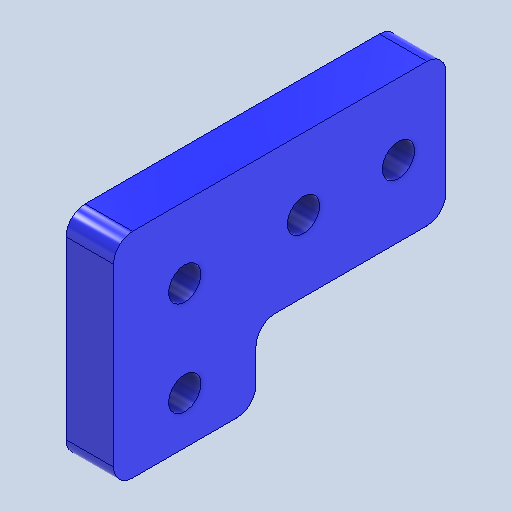
# Autodesk Inventor part: ball_loading_v1_Plate_ASP_F_2
Saved by Autodesk Inventor 2025.1 (Build 291241000, 241)
## iProperties
Created: 2024-11-12
Part Number: ball_loading_v1_Plate_ASP_F_2
Material: ABS プラスチック
Document SubType Name: Modeling
Designer: haruy
Density: 1.06 g/cm^3
Appearance: 青 - 壁塗料 - 光沢
Author: haruy
Autodesk Inventor part; units mm, degrees
ref_plane "YZ Plane" through (0, 0, 0) normal (1, 0, 0) x (0, 1, 0)
ref_plane "XZ Plane" through (0, 0, 0) normal (0, 1, 0) x (-1, 0, 0)
ref_plane "XY Plane" through (0, 0, 0) normal (0, 0, 1) x (1, 0, 0)
sketch "スケッチ1" plane through (0, 0, 0) normal (1, 0, 0) x (0, 1, 0)
  line L0 (-166.8338, 198.3583) -> (193.1662, 198.3583)
  line L1 (193.1662, 198.3583) -> (193.1662, 183.3583)
  line L2 (193.1662, 183.3583) -> (-166.8338, 183.3583)
  line L3 (-166.8338, 183.3583) -> (-166.8338, 198.3583)
  line L4 (-166.8338, 233.3583) -> (-181.8338, 233.3583)
  line L5 (-181.8338, 233.3583) -> (-181.8338, 5.8583)
  line L6 (-181.8338, 5.8583) -> (-166.8338, 5.8583)
  line L7 (-166.8338, 5.8583) -> (-166.8338, 233.3583)
  line L8 (-166.8338, 233.3583) -> (-181.8338, 233.3583)
  line L9 (-181.8338, 233.3583) -> (-181.8338, 218.3583)
  line L10 (-181.8338, 218.3583) -> (-166.8338, 218.3583)
  line L11 (-166.8338, 218.3583) -> (-166.8338, 233.3583)
  line L12 (-116.8338, 183.3583) -> (-101.8338, 183.3583)
  line L13 (-101.8338, 183.3583) -> (-101.8338, 5.8583)
  line L14 (-101.8338, 5.8583) -> (-116.8338, 5.8583)
  line L15 (-116.8338, 5.8583) -> (-116.8338, 183.3583)
  line L16 (193.1662, 183.3583) -> (178.1662, 183.3583)
  line L17 (178.1662, 183.3583) -> (178.1662, 5.8583)
  line L18 (178.1662, 5.8583) -> (193.1662, 5.8583)
  line L19 (193.1662, 5.8583) -> (193.1662, 183.3583)
  circle A0 centre (-141.8338, 138.3583) radius 12.5
  circle A1 centre (-141.8338, 98.3583) radius 18.75
  line L20 (193.1662, 5.8583) -> (-166.8338, 5.8583)
  line L21 (-181.8338, 158.3583) -> (-101.8338, 158.3583)
  line L22 (-101.8338, 78.3583) -> (-181.8338, 78.3583)
  circle A2 centre (-141.8338, 98.3583) radius 20
  line L23 (-124.3338, 198.3583) -> (-124.3338, 183.3583)
  line L24 (-101.8338, 183.3583) -> (-101.8338, 198.3583)
  line L25 (-146.8338, 198.3583) -> (-146.8338, 183.3583)
  line L26 (-166.8338, 205.8583) -> (-181.8338, 205.8583)
  line L27 (-166.8338, 175.8583) -> (-181.8338, 175.8583)
  circle A3 centre (158.1662, 138.3583) radius 12.5
  line L28 (193.1662, 163.3583) -> (178.1662, 163.3583)
  line L29 (170.6662, 198.3583) -> (170.6662, 183.3583)
  line L30 (-166.8338, -186.6417) -> (193.1662, -186.6417)
  line L31 (193.1662, -186.6417) -> (193.1662, -171.6417)
  line L32 (193.1662, -171.6417) -> (-166.8338, -171.6417)
  line L33 (-166.8338, -171.6417) -> (-166.8338, -186.6417)
  line L34 (-166.8338, -221.6417) -> (-181.8338, -221.6417)
  line L35 (-181.8338, -221.6417) -> (-181.8338, 5.8583)
  line L36 (-166.8338, 5.8583) -> (-166.8338, -221.6417)
  line L37 (-166.8338, -221.6417) -> (-181.8338, -221.6417)
  line L38 (-181.8338, -221.6417) -> (-181.8338, -206.6417)
  line L39 (-181.8338, -206.6417) -> (-166.8338, -206.6417)
  line L40 (-166.8338, -206.6417) -> (-166.8338, -221.6417)
  line L41 (-116.8338, -171.6417) -> (-101.8338, -171.6417)
  line L42 (-101.8338, -171.6417) -> (-101.8338, 5.8583)
  line L43 (-116.8338, 5.8583) -> (-116.8338, -171.6417)
  line L44 (193.1662, -171.6417) -> (178.1662, -171.6417)
  line L45 (178.1662, -171.6417) -> (178.1662, 5.8583)
  line L46 (193.1662, 5.8583) -> (193.1662, -171.6417)
  circle A4 centre (-141.8338, -126.6417) radius 12.5
  circle A5 centre (-141.8338, -86.6417) radius 18.75
  line L47 (-181.8338, -146.6417) -> (-101.8338, -146.6417)
  line L48 (-101.8338, -66.6417) -> (-181.8338, -66.6417)
  circle A6 centre (-141.8338, -86.6417) radius 20
  line L49 (-124.3338, -186.6417) -> (-124.3338, -171.6417)
  line L50 (-101.8338, -171.6417) -> (-101.8338, -186.6417)
  line L51 (-146.8338, -186.6417) -> (-146.8338, -171.6417)
  line L52 (-166.8338, -194.1417) -> (-181.8338, -194.1417)
  line L53 (-166.8338, -164.1417) -> (-181.8338, -164.1417)
  circle A7 centre (158.1662, -126.6417) radius 12.5
  line L54 (193.1662, -151.6417) -> (178.1662, -151.6417)
  line L55 (170.6662, -186.6417) -> (170.6662, -171.6417)
  line L56 (193.1662, 158.3583) -> (145.6662, 158.3583)
  line L57 (145.6662, 158.3583) -> (145.6662, 78.3583)
  line L58 (145.6662, 78.3583) -> (193.1662, 78.3583)
  line L59 (193.1662, 78.3583) -> (193.1662, 158.3583)
  line L60 (178.1662, 158.3583) -> (154.1437, 150.1934)
  line L61 (147.3229, 132.1397) -> (178.1662, 78.3583)
  circle A8 centre (-119.3338, 190.8583) radius 1.7
  circle A9 centre (-109.3338, 190.8583) radius 1.7
  circle A10 centre (-109.3338, 178.3583) radius 1.7
  circle A11 centre (-109.3338, 168.3583) radius 1.7
  line L62 (-101.8338, 163.3583) -> (-116.8338, 163.3583)
  point P0 (0, 0)
  point P1 (-174.3338, 200.8583)
  point P2 (-174.3338, 190.8583)
  point P3 (-174.3338, 180.8583)
  point P4 (-161.8338, 190.8583)
  point P5 (-151.8338, 190.8583)
  point P6 (185.6662, 178.3583)
  point P7 (185.6662, 168.3583)
  point P8 (185.6662, 190.8583)
  point P9 (175.6662, 190.8583)
  point P10 (-109.3338, 183.3583)
  point P11 (193.1662, 190.8583)
  point P12 (-109.3338, 98.3583)
  point P13 (-109.3338, 138.3583)
  point P14 (-174.3338, 138.3583)
  point P15 (-174.3338, 98.3583)
  point P16 (-174.3338, -86.6417)
  point P17 (-109.3338, -86.6417)
  point P18 (-109.3338, -126.6417)
  point P19 (-174.3338, -126.6417)
  point P20 (-174.3338, -169.1417)
  point P21 (-174.3338, -179.1417)
  point P22 (-174.3338, -189.1417)
  point P23 (-161.8338, -179.1417)
  point P24 (-151.8338, -179.1417)
  point P25 (-119.3338, -179.1417)
  point P26 (-109.3338, -179.1417)
  point P27 (-109.3338, -166.6417)
  point P28 (-109.3338, -156.6417)
  point P29 (175.6662, -179.1417)
  point P30 (185.6662, -179.1417)
  point P31 (185.6662, -166.6417)
  point P32 (185.6662, -156.6417)
  point P33 (185.6662, 138.3583)
  point P34 (185.6662, 98.3583)
  point P35 (178.1662, 94.6083)
  point P36 (185.6662, -86.6417)
  point P37 (185.6662, -126.6417)
  point P38 (-116.8338, 158.3583)
  dimension "d0" = 7.5
  dimension "d1" = 7.5
  dimension "d2" = 7.5
  dimension "d3" = 7.5
  dimension "d4" = 10
  dimension "d5" = 10
  dimension "d6" = 5
  dimension "d7" = 10
  dimension "d8" = 7.5
  dimension "d9" = 7.5
  dimension "d10" = 7.5
  dimension "d11" = 10
  dimension "d12" = 7.5
  dimension "d13" = 7.5
  dimension "d14" = 5
  dimension "d15" = 10
  dimension "d16" = 7.5
  dimension "d17" = 7.5
  dimension "d18" = 7.5
  dimension "d19" = 10
  dimension "d20" = 7.5
  dimension "d21" = 7.5
  dimension "d22" = 5
  dimension "d23" = 10
  dimension "d24" = 7.5
  dimension "d25" = 7.5
  dimension "d26" = 20
  dimension "d27" = 20
  dimension "d28" = 7.5
  dimension "d29" = 7.5
  dimension "d30" = 20
  dimension "d31" = 7.5
  dimension "d32" = 7.5
  dimension "d33" = 20
  dimension "d34" = 3.4
  dimension "d35" = 3.4
  dimension "d36" = 3.4
  dimension "d37" = 3.4
  dimension "d41" = 5
  constraints: 126 end point, 19 symmetric about line, 12 centre point, 4 coincident, 2 midpoint, 2 point on line, 1 perpendicular
  measures "d0" distance from line of L3 point (-174.334, 190.858)
  measures "d1" distance from line of point (-174.334, 200.858) L7
  measures "d2" distance from line of L7 point (-174.334, 180.858)
  measures "d3" distance from line of L2 point (-174.334, 190.858)
  measures "d4" distance of point (-174.334, 200.858) point (-174.334, 190.858)
  measures "d5" distance of point (-174.334, 180.858) point (-174.334, 190.858)
  measures "d6" distance from line of point (-161.834, 190.858) L3
  measures "d7" distance of point (-151.834, 190.858) point (-161.834, 190.858)
  measures "d8" distance from line of point (-161.834, 190.858) L0
  measures "d9" distance from line of L2 point (-151.834, 190.858)
  measures "d10" distance from line of point (-119.334, 190.858) L0
  measures "d11" distance of point (-109.334, 190.858) point (-119.334, 190.858)
  measures "d12" distance from line of L24 point (-109.334, 190.858)
  measures "d13" distance from line of L12 point (-109.334, 190.858)
  measures "d14" distance of point (-109.334, 178.358) point (-109.334, 183.358)
  measures "d15" distance of point (-109.334, 168.358) point (-109.334, 178.358)
  measures "d16" distance from line of point (-109.334, 178.358) L15
  measures "d17" distance from line of point (-109.334, 168.358) L15
  measures "d18" distance of point (193.166, 190.858) point (185.666, 190.858)
  measures "d19" distance of point (175.666, 190.858) point (185.666, 190.858)
  measures "d20" distance from line of point (175.666, 190.858) L0
  measures "d21" distance from line of L0 point (185.666, 190.858)
  measures "d22" distance from line of point (185.666, 178.358) L16
  measures "d23" distance of point (185.666, 168.358) point (185.666, 178.358)
  measures "d24" distance from line of L19 point (185.666, 178.358)
  measures "d25" distance from line of L19 point (185.666, 168.358)
  measures "d26" distance from line of L21 point (-109.334, 138.358)
  measures "d27" distance from line of L22 point (-109.334, 98.358)
  measures "d28" distance from line of L15 point (-109.334, 98.358)
  measures "d29" distance from line of L15 point (-109.334, 138.358)
  measures "d30" distance from line of L21 point (-174.334, 138.358)
  measures "d31" distance from line of point (-174.334, 138.358) L5
  measures "d32" distance from line of point (-174.334, 98.358) L5
  measures "d33" distance from line of L22 point (-174.334, 98.358)
  measures "d34" diameter of A8
  measures "d35" diameter of A9
  measures "d36" diameter of A10
  measures "d37" diameter of A11
  measures "d41" distance from line of A11.centre L62
extrude "押し出し1" add sketch "スケッチ1" along normal blind 5 contours L0 L24 L2 L23 | L13 L62 L15 L2
fillet "フィレット1" radius 2 6 edges at (2.5, -101.8338, 198.3583) (2.5, -124.3338, 198.3583) (2.5, -124.3338, 183.3583) (2.5, -116.8338, 183.3583) (2.5, -116.8338, 163.3583) (2.5, -101.8338, 163.3583)
equation "\"d1\" = d0"
equation "\"d2\" = d0"
equation "\"d3\" = d0"
equation "\"d8\" = d0"
equation "\"d9\" = d0"
equation "\"d10\" = d0"
equation "\"d12\" = d0"
equation "\"d13\" = d0"
equation "\"d16\" = d0"
equation "\"d17\" = d0"
equation "\"d20\" = d18"
equation "\"d21\" = d18"
equation "\"d24\" = d18"
equation "\"d25\" = d18"
equation "\"d32\" = d31"
equation "\"d33\" = d30"
